Autodesk Inventor part; units mm, degrees
(part 3 of 5)
  line L98 (0, 22) -> (0, -22) construction
  circle A131 centre (-90.3659, 45.1111) radius 1.6
  circle A132 centre (-45.1111, 90.3659) radius 1.6
  circle A133 centre (90.3659, -45.1111) radius 1.6
  circle A134 centre (45.1111, -90.3659) radius 1.6
  circle A135 centre (90.3659, 45.1111) radius 1.6
  circle A136 centre (45.1111, 90.3659) radius 1.6
  line L99 (41.3657, 27.2236) -> (27.2236, 41.3657) construction
  line L100 (34.2947, 34.2947) -> (55.1543, 55.1543) construction
  line L101 (46.669, 63.6396) -> (63.6396, 46.669) construction
  line L102 (0, 0) -> (0, -61.2072) construction
  circle A137 centre (0, -54) radius 1.6
  arc A138 (3.4868, -52.0398) -> (-3.4868, -52.0398) centre (0, -54) ccw
  line L103 (-0.6161, -51.9466) -> (-14.5119, -56.4463) construction
  line L104 (-5.1776, -53.4237) -> (-14.5119, -56.4463) construction
  line L105 (14.5119, -56.4463) -> (0.6161, -51.9466) construction
  line L106 (5.1776, -53.4237) -> (14.5119, -56.4463) construction
  arc A139 (0, -58) -> (3.8733, -53.0013) centre (0, -54) ccw construction
  arc A140 (-3.8733, -53.0013) -> (0, -58) centre (0, -54) ccw construction
  arc A141 (-5.1776, -53.4237) -> (-3.4868, -52.0398) centre (-6.1018, -50.5696) ccw
  arc A142 (3.4868, -52.0398) -> (5.1776, -53.4237) centre (6.1018, -50.5696) ccw
  line L107 (5.1776, -53.4237) -> (3.794, -57.2809)
  line L108 (3.794, -57.2809) -> (-2.6441, -58)
  line L109 (-2.6441, -58) -> (-5.1776, -53.4237)
  dimension "d114" = 3.2
  dimension "d117" = 64
  dimension "d118" = 3.2
  dimension "d119" = 54
  dimension "d120" = 8
  dimension "d121" = 3
  constraints: 20 end point, 15 centre point, 14 point on circle, 7 symmetric about line, 6 point on line, 4 midpoint, 4 tangent, 2 coincident, 2 collinear, 2 vertical, 1 equal radius, 1 horizontal, 7 other
  measures "d114" diameter of A129
  measures "d117" distance of A135.centre A136.centre
  measures "d118" diameter of A137
  measures "d119" distance of A137.centre point (0, 0)
  measures "d120" diameter of A138
  measures "d121" radius of A141
extrude "Выдавливание9" cut sketch "Эскиз6" against normal blind 10 contours A129 | A130 | A131 | A132 | A133 | A134 | A135 | A136 | A137
extrude "Выдавливание10" add sketch "Эскиз6" against normal blind 2 contours A142 L107 L108 L109 A141 A138
sketch "Эскиз7" plane through (0, 2, 0) normal (0, 1, 0) x (1, 0, 0)
  line L0 (-25, -33.1335) -> (25, -33.1335) construction
  line L1 (25, -33.1335) -> (25, -43.1335) construction
  line L2 (25, -43.1335) -> (-25, -43.1335) construction
  line L3 (-25, -43.1335) -> (-25, -33.1335) construction
  line L4 (0, 0) -> (0, -69.4501) construction
  circle A0 centre (21.9203, -43.1335) radius 1.6 construction
  circle A1 centre (-21.9203, -43.1335) radius 1.6 construction
  dimension "d124" = 50
  dimension "d125" = 10
  constraints: 10 end point, 2 parallel, 1 horizontal, 1 perpendicular, 1 point on line, 1 vertical, 1 other
  measures "d124" distance of L1.end L2.end
  measures "d125" distance of L0.end L1.end
sketch "Эскиз8" plane through (0, 0, 0) normal (0, -1, 0) x (1, 0, 0)
  circle A0 centre (0, 54) radius 1.6 construction
  line L0 (14.5119, 56.4463) -> (5.1776, 53.4237) construction
  arc A1 (15.1585, 56.5907) -> (14.5119, 56.4463) centre (15.6055, 53.069) ccw construction
  line L1 (20.596, 57.2809) -> (15.1585, 56.5907) construction
  line L2 (20.596, 57.2809) -> (26.2105, 51.6664) construction
  line L3 (26.2105, 51.6664) -> (21.6698, 47.1257) construction
  arc A2 (21.6698, 47.1257) -> (17.9282, 43.384) centre (21.9203, 43.1335) ccw construction
  line L4 (17.9282, 43.384) -> (1.4142, 26.8701) construction
  arc A3 (-1.4142, 26.8701) -> (1.4142, 26.8701) centre (0, 28.2843) ccw construction
  line L5 (-1.4142, 26.8701) -> (-17.9282, 43.384) construction
  arc A4 (-17.9282, 43.384) -> (-21.6698, 47.1257) centre (-21.9203, 43.1335) ccw construction
  line L6 (-21.6698, 47.1257) -> (-26.2105, 51.6664) construction
  line L7 (-26.2105, 51.6664) -> (-20.596, 57.2809) construction
  line L8 (-15.1585, 56.5907) -> (-20.596, 57.2809) construction
  arc A5 (-14.5119, 56.4463) -> (-15.1585, 56.5907) centre (-15.6055, 53.069) ccw construction
  line L9 (-5.1776, 53.4237) -> (-14.5119, 56.4463) construction
  arc A6 (-3.4868, 52.0398) -> (-5.1776, 53.4237) centre (-6.1018, 50.5696) ccw construction
  arc A7 (-3.4868, 52.0398) -> (3.4868, 52.0398) centre (0, 54) ccw construction
  arc A8 (5.1776, 53.4237) -> (3.4868, 52.0398) centre (6.1018, 50.5696) ccw construction
  circle A9 centre (45.1111, 90.3659) radius 1.6 construction
  circle A10 centre (-45.1111, -90.3659) radius 1.6 construction
  circle A11 centre (-90.3659, -45.1111) radius 1.6 construction
  circle A12 centre (90.3659, 45.1111) radius 1.6 construction
  circle A13 centre (-45.1111, 90.3659) radius 1.6 construction
  circle A14 centre (45.1111, -90.3659) radius 1.6 construction
  circle A15 centre (-90.3659, 45.1111) radius 1.6 construction
  circle A16 centre (90.3659, -45.1111) radius 1.6 construction
  circle A17 centre (101, 0) radius 1.6 construction
  circle A18 centre (-101, 0) radius 1.6 construction
  arc A19 (-93.0503, 48.6481) -> (-93.0503, -48.6481) centre (0, 0) ccw construction
  arc A20 (-93.0503, -48.6481) -> (-88.2704, -49.3795) centre (-90.3917, -47.2582) ccw construction
  line L10 (-85.2064, -46.3155) -> (-88.2704, -49.3795) construction
  arc A21 (-73.8927, -46.3155) -> (-85.2064, -46.3155) centre (-79.5495, -51.9723) ccw construction
  line L11 (-46.3155, -73.8927) -> (-73.8927, -46.3155) construction
  arc A22 (-46.3155, -85.2064) -> (-46.3155, -73.8927) centre (-51.9723, -79.5495) ccw construction
  line L12 (-49.3795, -88.2704) -> (-46.3155, -85.2064) construction
  arc A23 (-49.3795, -88.2704) -> (-48.6481, -93.0503) centre (-47.2582, -90.3917) ccw construction
  arc A24 (-48.6481, -93.0503) -> (-11.8382, -104.3305) centre (0, 0) ccw construction
  arc A25 (-11.8382, -104.3305) -> (-8.5, -101.3496) centre (-11.5, -101.3496) ccw construction
  line L13 (-8.5, -101.3496) -> (-8.5, -90.5) construction
  arc A26 (-7, -89) -> (-8.5, -90.5) centre (-7, -90.5) ccw construction
  line L14 (-7, -89) -> (7, -89) construction
  arc A27 (8.5, -90.5) -> (7, -89) centre (7, -90.5) ccw construction
  line L15 (8.5, -90.5) -> (8.5, -101.3496) construction
  arc A28 (8.5, -101.3496) -> (11.8382, -104.3305) centre (11.5, -101.3496) ccw construction
  arc A29 (11.8382, -104.3305) -> (48.6481, -93.0503) centre (0, 0) ccw construction
  arc A30 (48.6481, -93.0503) -> (49.3795, -88.2704) centre (47.2582, -90.3917) ccw construction
  line L16 (46.3155, -85.2064) -> (49.3795, -88.2704) construction
  arc A31 (46.3155, -73.8927) -> (46.3155, -85.2064) centre (51.9723, -79.5495) ccw construction
  line L17 (73.8927, -46.3155) -> (46.3155, -73.8927) construction
  arc A32 (85.2064, -46.3155) -> (73.8927, -46.3155) centre (79.5495, -51.9723) ccw construction
  line L18 (88.2704, -49.3795) -> (85.2064, -46.3155) construction
  arc A33 (88.2704, -49.3795) -> (93.0503, -48.6481) centre (90.3917, -47.2582) ccw construction
  arc A34 (93.0503, -48.6481) -> (93.0503, 48.6481) centre (0, 0) ccw construction
  arc A35 (93.0503, 48.6481) -> (88.2704, 49.3795) centre (90.3917, 47.2582) ccw construction
  line L19 (85.2064, 46.3155) -> (88.2704, 49.3795) construction
  arc A36 (73.8927, 46.3155) -> (85.2064, 46.3155) centre (79.5495, 51.9723) ccw construction
  line L20 (46.3155, 73.8927) -> (73.8927, 46.3155) construction
  arc A37 (46.3155, 85.2064) -> (46.3155, 73.8927) centre (51.9723, 79.5495) ccw construction
  line L21 (49.3795, 88.2704) -> (46.3155, 85.2064) construction
  arc A38 (49.3795, 88.2704) -> (48.6481, 93.0503) centre (47.2582, 90.3917) ccw construction
  arc A39 (48.6481, 93.0503) -> (45.42, 94.668) centre (0, 0) ccw construction
  arc A40 (45.42, 94.668) -> (43.0355, 94.1655) centre (44.5548, 92.8648) ccw construction
  line L22 (18.3802, 65.3664) -> (43.0355, 94.1655) construction
  arc A41 (17.477, 64.7643) -> (18.3802, 65.3664) centre (16.8609, 66.6671) ccw construction
  line L23 (0.6161, 59.3045) -> (17.477, 64.7643) construction
  arc A42 (-0.6161, 59.3045) -> (0.6161, 59.3045) centre (0, 61.2072) ccw construction
  line L24 (-17.477, 64.7643) -> (-0.6161, 59.3045) construction
  arc A43 (-18.3802, 65.3664) -> (-17.477, 64.7643) centre (-16.8609, 66.6671) ccw construction
  line L25 (-43.0355, 94.1655) -> (-18.3802, 65.3664) construction
  arc A44 (-43.0355, 94.1655) -> (-45.42, 94.668) centre (-44.5548, 92.8648) ccw construction
  arc A45 (-45.42, 94.668) -> (-48.6481, 93.0503) centre (0, 0) ccw construction
  arc A46 (-48.6481, 93.0503) -> (-49.3795, 88.2704) centre (-47.2582, 90.3917) ccw construction
  line L26 (-46.3155, 85.2064) -> (-49.3795, 88.2704) construction
  arc A47 (-46.3155, 73.8927) -> (-46.3155, 85.2064) centre (-51.9723, 79.5495) ccw construction
  line L27 (-73.8927, 46.3155) -> (-46.3155, 73.8927) construction
  arc A48 (-85.2064, 46.3155) -> (-73.8927, 46.3155) centre (-79.5495, 51.9723) ccw construction
  line L28 (-88.2704, 49.3795) -> (-85.2064, 46.3155) construction
  arc A49 (-88.2704, 49.3795) -> (-93.0503, 48.6481) centre (-90.3917, 47.2582) ccw construction
  arc A50 (90.4395, -37.7453) -> (97.9653, -2.6059) centre (0, 0) ccw construction
  arc A51 (87.1795, -38.3892) -> (90.4395, -37.7453) centre (88.5938, -36.975) ccw construction
  line L29 (83.085, -34.2947) -> (87.1795, -38.3892) construction
  arc A52 (83.085, -34.2947) -> (76.014, -34.2947) centre (79.5495, -37.8302) ccw construction
  line L30 (67.8823, -42.4264) -> (76.014, -34.2947) construction
  line L31 (67.8823, -42.4264) -> (47.1257, -21.6698) construction
  arc A53 (47.1257, -21.6698) -> (43.384, -17.9282) centre (43.1335, -21.9203) ccw construction
  line L32 (43.384, -17.9282) -> (26.8701, -1.4142) construction
  arc A54 (26.8701, 1.4142) -> (26.8701, -1.4142) centre (28.2843, 0) ccw construction
  line L33 (26.8701, 1.4142) -> (43.384, 17.9282) construction
  arc A55 (43.384, 17.9282) -> (47.1257, 21.6698) centre (43.1335, 21.9203) ccw construction
  line L34 (47.1257, 21.6698) -> (67.8823, 42.4264) construction
  line L35 (76.014, 34.2947) -> (67.8823, 42.4264) construction
  arc A56 (76.014, 34.2947) -> (83.085, 34.2947) centre (79.5495, 37.8302) ccw construction
  line L36 (87.1795, 38.3892) -> (83.085, 34.2947) construction
  arc A57 (90.4395, 37.7453) -> (87.1795, 38.3892) centre (88.5938, 36.975) ccw construction
  arc A58 (97.9653, 2.6059) -> (90.4395, 37.7453) centre (0, 0) ccw construction
  arc A59 (97.9653, 2.6059) -> (97.9653, -2.6059) centre (101, 0) ccw construction
  line L37 (29.746, 55.2019) -> (24.3148, 60.6331) construction
  line L38 (24.842, 61.8893) -> (24.3148, 60.6331) construction
  arc A60 (25.4187, 62.8242) -> (24.842, 61.8893) centre (28.1154, 60.5155) ccw construction
  line L39 (34.1909, 73.0707) -> (25.4187, 62.8242) construction
  arc A61 (37.1244, 73.1843) -> (34.1909, 73.0707) centre (35.7102, 71.7701) ccw construction
  line L40 (42.4264, 67.8823) -> (37.1244, 73.1843) construction
  line L41 (42.4264, 67.8823) -> (29.746, 55.2019) construction
  arc A62 (14.5, -93.3742) -> (18.0526, -96.3229) centre (17.5, -93.3742) ccw construction
  line L42 (14.5, -93.3742) -> (14.5, -87) construction
  arc A63 (14.5, -87) -> (11.5, -84) centre (11.5, -87) ccw construction
  line L43 (11.5, -84) -> (-11.5, -84) construction
  arc A64 (-11.5, -84) -> (-14.5, -87) centre (-11.5, -87) ccw construction
  line L44 (-14.5, -87) -> (-14.5, -93.3742) construction
  arc A65 (-18.0526, -96.3229) -> (-14.5, -93.3742) centre (-17.5, -93.3742) ccw construction
  arc A66 (-37.7453, -90.4395) -> (-18.0526, -96.3229) centre (0, 0) ccw construction
  arc A67 (-38.3892, -87.1795) -> (-37.7453, -90.4395) centre (-36.975, -88.5938) ccw construction
  line L45 (-34.2947, -83.085) -> (-38.3892, -87.1795) construction
  arc A68 (-34.2947, -83.085) -> (-34.2947, -76.014) centre (-37.8302, -79.5495) ccw construction
  line L46 (-42.4264, -67.8823) -> (-34.2947, -76.014) construction
  line L47 (-42.4264, -67.8823) -> (-21.6698, -47.1257) construction
  arc A69 (-21.6698, -47.1257) -> (-17.9282, -43.384) centre (-21.9203, -43.1335) ccw construction
  line L48 (-17.9282, -43.384) -> (-1.4142, -26.8701) construction
  arc A70 (1.4142, -26.8701) -> (-1.4142, -26.8701) centre (0, -28.2843) ccw construction
  line L49 (1.4142, -26.8701) -> (17.9282, -43.384) construction
  arc A71 (17.9282, -43.384) -> (21.6698, -47.1257) centre (21.9203, -43.1335) ccw construction
  line L50 (21.6698, -47.1257) -> (42.4264, -67.8823) construction
  line L51 (34.2947, -76.014) -> (42.4264, -67.8823) construction
  arc A72 (34.2947, -76.014) -> (34.2947, -83.085) centre (37.8302, -79.5495) ccw construction
  line L52 (38.3892, -87.1795) -> (34.2947, -83.085) construction
  arc A73 (37.7453, -90.4395) -> (38.3892, -87.1795) centre (36.975, -88.5938) ccw construction
  arc A74 (18.0526, -96.3229) -> (37.7453, -90.4395) centre (0, 0) ccw construction
  line L53 (63.6396, 46.669) -> (46.669, 63.6396) construction
  line L54 (63.6396, 46.669) -> (44.1942, 27.2236) construction
  arc A75 (41.3657, 27.2236) -> (44.1942, 27.2236) centre (42.78, 28.6378) ccw construction
  line L55 (41.3657, 27.2236) -> (27.2236, 41.3657) construction
  arc A76 (27.2236, 44.1942) -> (27.2236, 41.3657) centre (28.6378, 42.78) ccw construction
  line L56 (27.2236, 44.1942) -> (46.669, 63.6396) construction
  line L57 (46.669, -63.6396) -> (63.6396, -46.669) construction
  line L58 (46.669, -63.6396) -> (27.2236, -44.1942) construction
  arc A77 (27.2236, -41.3657) -> (27.2236, -44.1942) centre (28.6378, -42.78) ccw construction
  line L59 (27.2236, -41.3657) -> (41.3657, -27.2236) construction
  arc A78 (44.1942, -27.2236) -> (41.3657, -27.2236) centre (42.78, -28.6378) ccw construction
  line L60 (44.1942, -27.2236) -> (63.6396, -46.669) construction
  line L61 (-63.6396, -46.669) -> (-46.669, -63.6396) construction
  line L62 (-63.6396, -46.669) -> (-44.1942, -27.2236) construction
  arc A79 (-41.3657, -27.2236) -> (-44.1942, -27.2236) centre (-42.78, -28.6378) ccw construction
  line L63 (-41.3657, -27.2236) -> (-27.2236, -41.3657) construction
  arc A80 (-27.2236, -44.1942) -> (-27.2236, -41.3657) centre (-28.6378, -42.78) ccw construction
  line L64 (-27.2236, -44.1942) -> (-46.669, -63.6396) construction
  line L65 (-46.669, 63.6396) -> (-63.6396, 46.669) construction
  line L66 (-46.669, 63.6396) -> (-27.2236, 44.1942) construction
  arc A81 (-27.2236, 41.3657) -> (-27.2236, 44.1942) centre (-28.6378, 42.78) ccw construction
  line L67 (-27.2236, 41.3657) -> (-41.3657, 27.2236) construction
  arc A82 (-44.1942, 27.2236) -> (-41.3657, 27.2236) centre (-42.78, 28.6378) ccw construction
  line L68 (-44.1942, 27.2236) -> (-63.6396, 46.669) construction
  arc A83 (7.7166, 24.6871) -> (8.4003, 21.4111) centre (9.1308, 23.2729) ccw construction
  line L69 (7.7166, 24.6871) -> (20.8597, 37.8302) construction
  arc A84 (23.6881, 37.8302) -> (20.8597, 37.8302) centre (22.2739, 36.416) ccw construction
  line L70 (23.6881, 37.8302) -> (37.8302, 23.6881) construction
  arc A85 (37.8302, 20.8597) -> (37.8302, 23.6881) centre (36.416, 22.2739) ccw construction
  line L71 (37.8302, 20.8597) -> (24.6871, 7.7166) construction
  arc A86 (21.4111, 8.4003) -> (24.6871, 7.7166) centre (23.2729, 9.1308) ccw construction
  arc A87 (21.4111, 8.4003) -> (8.4003, 21.4111) centre (0, 0) ccw construction
  circle A88 centre (-21.9203, -43.1335) radius 1.6 construction
  arc A89 (-21.4111, -8.4003) -> (-24.6871, -7.7166) centre (-23.2729, -9.1308) ccw construction
  arc A90 (-21.4111, -8.4003) -> (-8.4003, -21.4111) centre (0, 0) ccw construction
  arc A91 (-7.7166, -24.6871) -> (-8.4003, -21.4111) centre (-9.1308, -23.2729) ccw construction
  line L72 (-7.7166, -24.6871) -> (-20.8597, -37.8302) construction
  arc A92 (-23.6881, -37.8302) -> (-20.8597, -37.8302) centre (-22.2739, -36.416) ccw construction
  line L73 (-23.6881, -37.8302) -> (-37.8302, -23.6881) construction
  arc A93 (-37.8302, -20.8597) -> (-37.8302, -23.6881) centre (-36.416, -22.2739) ccw construction
  line L74 (-37.8302, -20.8597) -> (-24.6871, -7.7166) construction
  line L75 (24.6871, -7.7166) -> (37.8302, -20.8597) construction
  arc A94 (37.8302, -23.6881) -> (37.8302, -20.8597) centre (36.416, -22.2739) ccw construction
  line L76 (37.8302, -23.6881) -> (23.6881, -37.8302) construction
  arc A95 (20.8597, -37.8302) -> (23.6881, -37.8302) centre (22.2739, -36.416) ccw construction
  line L77 (20.8597, -37.8302) -> (7.7166, -24.6871) construction
  arc A96 (8.4003, -21.4111) -> (7.7166, -24.6871) centre (9.1308, -23.2729) ccw construction
  arc A97 (8.4003, -21.4111) -> (21.4111, -8.4003) centre (0, 0) ccw construction
  arc A98 (24.6871, -7.7166) -> (21.4111, -8.4003) centre (23.2729, -9.1308) ccw construction
  circle A99 centre (21.9203, 43.1335) radius 1.6 construction
  line L78 (-37.8302, 23.6881) -> (-23.6881, 37.8302) construction
  arc A100 (-20.8597, 37.8302) -> (-23.6881, 37.8302) centre (-22.2739, 36.416) ccw construction
  line L79 (-20.8597, 37.8302) -> (-7.7166, 24.6871) construction
  arc A101 (-8.4003, 21.4111) -> (-7.7166, 24.6871) centre (-9.1308, 23.2729) ccw construction
  arc A102 (-8.4003, 21.4111) -> (-21.4111, 8.4003) centre (0, 0) ccw construction
  arc A103 (-24.6871, 7.7166) -> (-21.4111, 8.4003) centre (-23.2729, 9.1308) ccw construction
  line L80 (-24.6871, 7.7166) -> (-37.8302, 20.8597) construction
  arc A104 (-37.8302, 23.6881) -> (-37.8302, 20.8597) centre (-36.416, 22.2739) ccw construction
  circle A105 centre (-43.1335, 21.9203) radius 1.6 construction
  circle A106 centre (43.1335, -21.9203) radius 1.6 construction
  circle A107 centre (21.9203, -43.1335) radius 1.6 construction
  circle A108 centre (-21.9203, 43.1335) radius 1.6 construction
  circle A109 centre (-43.1335, -21.9203) radius 1.6 construction
  circle A110 centre (0, 0) radius 18 construction
  circle A111 centre (43.1335, 21.9203) radius 1.6 construction
  circle A112 centre (0, -22) radius 1.6 construction
  circle A113 centre (-22, 0) radius 1.6 construction
  circle A114 centre (0, 22) radius 1.6 construction
  circle A115 centre (22, 0) radius 1.6 construction
  circle A116 centre (-37.8302, -79.5495) radius 1.6 construction
  circle A117 centre (-79.5495, -37.8302) radius 1.6 construction
  circle A118 centre (-79.5495, 37.8302) radius 1.6 construction
  circle A119 centre (79.5495, 37.8302) radius 1.6 construction
  circle A120 centre (37.8302, -79.5495) radius 1.6 construction
  circle A121 centre (79.5495, -37.8302) radius 1.6 construction
  circle A122 centre (-20.5578, 60.8546) radius 1.55 construction
  circle A123 centre (20.5578, 60.8546) radius 1.55 construction
  circle A124 centre (37.8302, 79.5495) radius 1.6 construction
  circle A125 centre (-37.8302, 79.5495) radius 1.6 construction
  line L81 (-24.3148, 60.6331) -> (-29.746, 55.2019) construction
  line L82 (-29.746, 55.2019) -> (-42.4264, 67.8823) construction
  line L83 (-37.1244, 73.1843) -> (-42.4264, 67.8823) construction
  arc A126 (-34.1909, 73.0707) -> (-37.1244, 73.1843) centre (-35.7102, 71.7701) ccw construction
  line L84 (-25.4187, 62.8242) -> (-34.1909, 73.0707) construction
  arc A127 (-24.842, 61.8893) -> (-25.4187, 62.8242) centre (-28.1154, 60.5155) ccw construction
  line L85 (-24.3148, 60.6331) -> (-24.842, 61.8893) construction
  arc A128 (-90.4395, 37.7453) -> (-97.9653, 2.6059) centre (0, 0) ccw construction
  arc A129 (-87.1795, 38.3892) -> (-90.4395, 37.7453) centre (-88.5938, 36.975) ccw construction
  line L86 (-83.085, 34.2947) -> (-87.1795, 38.3892) construction
  arc A130 (-83.085, 34.2947) -> (-76.014, 34.2947) centre (-79.5495, 37.8302) ccw construction
  line L87 (-67.8823, 42.4264) -> (-76.014, 34.2947) construction
  line L88 (-67.8823, 42.4264) -> (-47.1257, 21.6698) construction
  arc A131 (-47.1257, 21.6698) -> (-43.384, 17.9282) centre (-43.1335, 21.9203) ccw construction
  line L89 (-43.384, 17.9282) -> (-26.8701, 1.4142) construction
  arc A132 (-26.8701, -1.4142) -> (-26.8701, 1.4142) centre (-28.2843, 0) ccw construction
  line L90 (-26.8701, -1.4142) -> (-43.384, -17.9282) construction
  arc A133 (-43.384, -17.9282) -> (-47.1257, -21.6698) centre (-43.1335, -21.9203) ccw construction
  line L91 (-47.1257, -21.6698) -> (-67.8823, -42.4264) construction
  line L92 (-76.014, -34.2947) -> (-67.8823, -42.4264) construction
  arc A134 (-76.014, -34.2947) -> (-83.085, -34.2947) centre (-79.5495, -37.8302) ccw construction
  line L93 (-87.1795, -38.3892) -> (-83.085, -34.2947) construction
  arc A135 (-90.4395, -37.7453) -> (-87.1795, -38.3892) centre (-88.5938, -36.975) ccw construction
  arc A136 (-97.9653, -2.6059) -> (-90.4395, -37.7453) centre (0, 0) ccw construction
  arc A137 (-97.9653, -2.6059) -> (-97.9653, 2.6059) centre (-101, 0) ccw construction
  line L94 (19.5177, 122.3748) -> (96.2153, 45.6773) construction
  arc A138 (93.0503, 48.6481) -> (88.2704, 49.3795) centre (90.3917, 47.2582) ccw construction
  line L95 (-105.344, -36.5485) -> (-36.5776, -105.315) construction
  arc A139 (-49.3795, -88.2704) -> (-48.6481, -93.0503) centre (-47.2582, -90.3917) ccw construction
  arc A140 (-93.0503, -48.6481) -> (-88.2704, -49.3795) centre (-90.3917, -47.2582) ccw construction
  circle A141 centre (0, 54) radius 1.6 construction
  arc A142 (-93.0503, 48.6481) -> (-93.0503, -48.6481) centre (0, 0) ccw construction
  arc A143 (-88.2704, 49.3795) -> (-93.0503, 48.6481) centre (-90.3917, 47.2582) ccw construction
  line L96 (-88.2704, 49.3795) -> (-85.2064, 46.3155) construction
  arc A144 (-85.2064, 46.3155) -> (-73.8927, 46.3155) centre (-79.5495, 51.9723) ccw construction
  line L97 (-73.8927, 46.3155) -> (-46.3155, 73.8927) construction
  arc A145 (-46.3155, 73.8927) -> (-46.3155, 85.2064) centre (-51.9723, 79.5495) ccw construction
  line L98 (-46.3155, 85.2064) -> (-49.3795, 88.2704) construction
  arc A146 (-48.6481, 93.0503) -> (-49.3795, 88.2704) centre (-47.2582, 90.3917) ccw construction
  arc A147 (-45.42, 94.668) -> (-48.6481, 93.0503) centre (0, 0) ccw construction
  arc A148 (-43.0355, 94.1655) -> (-45.42, 94.668) centre (-44.5548, 92.8648) ccw construction
  line L99 (-43.0355, 94.1655) -> (-18.3802, 65.3664) construction
  arc A149 (-18.3802, 65.3664) -> (-17.477, 64.7643) centre (-16.8609, 66.6671) ccw construction
  line L100 (-17.477, 64.7643) -> (-0.6161, 59.3045) construction
  arc A150 (-0.6161, 59.3045) -> (0.6161, 59.3045) centre (0, 61.2072) ccw construction
  line L101 (0.6161, 59.3045) -> (17.477, 64.7643) construction
  arc A151 (17.477, 64.7643) -> (18.3802, 65.3664) centre (16.8609, 66.6671) ccw construction
  line L102 (18.3802, 65.3664) -> (43.0355, 94.1655) construction
  arc A152 (45.42, 94.668) -> (43.0355, 94.1655) centre (44.5548, 92.8648) ccw construction
  arc A153 (48.6481, 93.0503) -> (45.42, 94.668) centre (0, 0) ccw construction
  arc A154 (49.3795, 88.2704) -> (48.6481, 93.0503) centre (47.2582, 90.3917) ccw construction
  line L103 (49.3795, 88.2704) -> (46.3155, 85.2064) construction
  arc A155 (46.3155, 85.2064) -> (46.3155, 73.8927) centre (51.9723, 79.5495) ccw construction
  line L104 (46.3155, 73.8927) -> (73.8927, 46.3155) construction
  arc A156 (73.8927, 46.3155) -> (85.2064, 46.3155) centre (79.5495, 51.9723) ccw construction
  line L105 (85.2064, 46.3155) -> (88.2704, 49.3795) construction
  arc A157 (93.0503, 48.6481) -> (88.2704, 49.3795) centre (90.3917, 47.2582) ccw construction
  arc A158 (93.0503, -48.6481) -> (93.0503, 48.6481) centre (0, 0) ccw construction
  arc A159 (88.2704, -49.3795) -> (93.0503, -48.6481) centre (90.3917, -47.2582) ccw construction
  line L106 (88.2704, -49.3795) -> (85.2064, -46.3155) construction
  arc A160 (85.2064, -46.3155) -> (73.8927, -46.3155) centre (79.5495, -51.9723) ccw construction
  line L107 (73.8927, -46.3155) -> (46.3155, -73.8927) construction
  arc A161 (46.3155, -73.8927) -> (46.3155, -85.2064) centre (51.9723, -79.5495) ccw construction
  line L108 (46.3155, -85.2064) -> (49.3795, -88.2704) construction
  arc A162 (48.6481, -93.0503) -> (49.3795, -88.2704) centre (47.2582, -90.3917) ccw construction
  arc A163 (11.8382, -104.3305) -> (48.6481, -93.0503) centre (0, 0) ccw construction
  arc A164 (8.5, -101.3496) -> (11.8382, -104.3305) centre (11.5, -101.3496) ccw construction
  line L109 (8.5, -101.3496) -> (8.5, -90.5) construction
  arc A165 (8.5, -90.5) -> (7, -89) centre (7, -90.5) ccw construction
  line L110 (7, -89) -> (-7, -89) construction
  arc A166 (-7, -89) -> (-8.5, -90.5) centre (-7, -90.5) ccw construction
  line L111 (-8.5, -90.5) -> (-8.5, -101.3496) construction
  arc A167 (-11.8382, -104.3305) -> (-8.5, -101.3496) centre (-11.5, -101.3496) ccw construction
  arc A168 (-48.6481, -93.0503) -> (-11.8382, -104.3305) centre (0, 0) ccw construction
  arc A169 (-49.3795, -88.2704) -> (-48.6481, -93.0503) centre (-47.2582, -90.3917) ccw construction
  line L112 (-49.3795, -88.2704) -> (-46.3155, -85.2064) construction
  arc A170 (-46.3155, -85.2064) -> (-46.3155, -73.8927) centre (-51.9723, -79.5495) ccw construction
  line L113 (-46.3155, -73.8927) -> (-73.8927, -46.3155) construction
  arc A171 (-73.8927, -46.3155) -> (-85.2064, -46.3155) centre (-79.5495, -51.9723) ccw construction
  line L114 (-85.2064, -46.3155) -> (-88.2704, -49.3795) construction
  arc A172 (-93.0503, -48.6481) -> (-88.2704, -49.3795) centre (-90.3917, -47.2582) ccw construction
  arc A173 (-97.9653, -2.6059) -> (-90.4395, -37.7453) centre (0, 0) ccw construction
  arc A174 (-90.4395, -37.7453) -> (-87.1795, -38.3892) centre (-88.5938, -36.975) ccw construction
  line L115 (-87.1795, -38.3892) -> (-83.085, -34.2947) construction
  arc A175 (-76.014, -34.2947) -> (-83.085, -34.2947) centre (-79.5495, -37.8302) ccw construction
  line L116 (-76.014, -34.2947) -> (-67.8823, -42.4264) construction
  line L117 (-67.8823, -42.4264) -> (-47.1257, -21.6698) construction
  arc A176 (-43.384, -17.9282) -> (-47.1257, -21.6698) centre (-43.1335, -21.9203) ccw construction
  line L118 (-43.384, -17.9282) -> (-26.8701, -1.4142) construction
  arc A177 (-26.8701, -1.4142) -> (-26.8701, 1.4142) centre (-28.2843, 0) ccw construction
  line L119 (-26.8701, 1.4142) -> (-43.384, 17.9282) construction
  arc A178 (-47.1257, 21.6698) -> (-43.384, 17.9282) centre (-43.1335, 21.9203) ccw construction
  line L120 (-47.1257, 21.6698) -> (-67.8823, 42.4264) construction
  line L121 (-67.8823, 42.4264) -> (-76.014, 34.2947) construction
  arc A179 (-83.085, 34.2947) -> (-76.014, 34.2947) centre (-79.5495, 37.8302) ccw construction
  line L122 (-83.085, 34.2947) -> (-87.1795, 38.3892) construction
  arc A180 (-87.1795, 38.3892) -> (-90.4395, 37.7453) centre (-88.5938, 36.975) ccw construction
  arc A181 (-90.4395, 37.7453) -> (-97.9653, 2.6059) centre (0, 0) ccw construction
  arc A182 (-97.9653, -2.6059) -> (-97.9653, 2.6059) centre (-101, 0) ccw construction
  line L123 (29.746, 55.2019) -> (42.4264, 67.8823) construction
  line L124 (42.4264, 67.8823) -> (37.1244, 73.1843) construction
  arc A183 (37.1244, 73.1843) -> (34.1909, 73.0707) centre (35.7102, 71.7701) ccw construction
  line L125 (34.1909, 73.0707) -> (25.4187, 62.8242) construction
  arc A184 (25.4187, 62.8242) -> (24.842, 61.8893) centre (28.1154, 60.5155) ccw construction
  line L126 (24.842, 61.8893) -> (24.3148, 60.6331) construction
  line L127 (24.3148, 60.6331) -> (29.746, 55.2019) construction
  arc A185 (5.1776, 53.4237) -> (3.4868, 52.0398) centre (6.1018, 50.5696) ccw construction
  arc A186 (-3.4868, 52.0398) -> (3.4868, 52.0398) centre (0, 54) ccw construction
  arc A187 (-3.4868, 52.0398) -> (-5.1776, 53.4237) centre (-6.1018, 50.5696) ccw construction
  line L128 (-5.1776, 53.4237) -> (-14.5119, 56.4463) construction
  arc A188 (-14.5119, 56.4463) -> (-15.1585, 56.5907) centre (-15.6055, 53.069) ccw construction
  line L129 (-15.1585, 56.5907) -> (-20.596, 57.2809) construction
  line L130 (-20.596, 57.2809) -> (-26.2105, 51.6664) construction
  line L131 (-26.2105, 51.6664) -> (-21.6698, 47.1257) construction
  arc A189 (-17.9282, 43.384) -> (-21.6698, 47.1257) centre (-21.9203, 43.1335) ccw construction
  line L132 (-17.9282, 43.384) -> (-1.4142, 26.8701) construction
  arc A190 (-1.4142, 26.8701) -> (1.4142, 26.8701) centre (0, 28.2843) ccw construction
  line L133 (1.4142, 26.8701) -> (17.9282, 43.384) construction
  arc A191 (21.6698, 47.1257) -> (17.9282, 43.384) centre (21.9203, 43.1335) ccw construction
  line L134 (21.6698, 47.1257) -> (26.2105, 51.6664) construction
  line L135 (26.2105, 51.6664) -> (20.596, 57.2809) construction
  line L136 (20.596, 57.2809) -> (15.1585, 56.5907) construction
  arc A192 (15.1585, 56.5907) -> (14.5119, 56.4463) centre (15.6055, 53.069) ccw construction
  line L137 (14.5119, 56.4463) -> (5.1776, 53.4237) construction
  arc A193 (18.0526, -96.3229) -> (37.7453, -90.4395) centre (0, 0) ccw construction
  arc A194 (37.7453, -90.4395) -> (38.3892, -87.1795) centre (36.975, -88.5938) ccw construction
  line L138 (38.3892, -87.1795) -> (34.2947, -83.085) construction
  arc A195 (34.2947, -76.014) -> (34.2947, -83.085) centre (37.8302, -79.5495) ccw construction
  line L139 (34.2947, -76.014) -> (42.4264, -67.8823) construction
  line L140 (42.4264, -67.8823) -> (21.6698, -47.1257) construction
  arc A196 (17.9282, -43.384) -> (21.6698, -47.1257) centre (21.9203, -43.1335) ccw construction
  line L141 (17.9282, -43.384) -> (1.4142, -26.8701) construction
  arc A197 (1.4142, -26.8701) -> (-1.4142, -26.8701) centre (0, -28.2843) ccw construction
  line L142 (-1.4142, -26.8701) -> (-17.9282, -43.384) construction
  arc A198 (-21.6698, -47.1257) -> (-17.9282, -43.384) centre (-21.9203, -43.1335) ccw construction
  line L143 (-21.6698, -47.1257) -> (-42.4264, -67.8823) construction
  line L144 (-42.4264, -67.8823) -> (-34.2947, -76.014) construction
  arc A199 (-34.2947, -83.085) -> (-34.2947, -76.014) centre (-37.8302, -79.5495) ccw construction
  line L145 (-34.2947, -83.085) -> (-38.3892, -87.1795) construction
  arc A200 (-38.3892, -87.1795) -> (-37.7453, -90.4395) centre (-36.975, -88.5938) ccw construction
  arc A201 (-37.7453, -90.4395) -> (-18.0526, -96.3229) centre (0, 0) ccw construction
  arc A202 (-18.0526, -96.3229) -> (-14.5, -93.3742) centre (-17.5, -93.3742) ccw construction
  line L146 (-14.5, -93.3742) -> (-14.5, -87) construction
  arc A203 (-11.5, -84) -> (-14.5, -87) centre (-11.5, -87) ccw construction
  line L147 (-11.5, -84) -> (11.5, -84) construction
  arc A204 (14.5, -87) -> (11.5, -84) centre (11.5, -87) ccw construction
  line L148 (14.5, -87) -> (14.5, -93.3742) construction
  arc A205 (14.5, -93.3742) -> (18.0526, -96.3229) centre (17.5, -93.3742) ccw construction
  line L149 (63.6396, -46.669) -> (44.1942, -27.2236) construction
  arc A206 (44.1942, -27.2236) -> (41.3657, -27.2236) centre (42.78, -28.6378) ccw construction
  line L150 (41.3657, -27.2236) -> (27.2236, -41.3657) construction
  arc A207 (27.2236, -41.3657) -> (27.2236, -44.1942) centre (28.6378, -42.78) ccw construction
  line L151 (27.2236, -44.1942) -> (46.669, -63.6396) construction
  line L152 (46.669, -63.6396) -> (63.6396, -46.669) construction
  circle A208 centre (-37.8302, 79.5495) radius 1.6 construction
  circle A209 centre (37.8302, 79.5495) radius 1.6 construction
  circle A210 centre (20.5578, 60.8546) radius 1.55 construction
  circle A211 centre (-20.5578, 60.8546) radius 1.55 construction
  circle A212 centre (79.5495, -37.8302) radius 1.6 construction
  circle A213 centre (37.8302, -79.5495) radius 1.6 construction
  circle A214 centre (79.5495, 37.8302) radius 1.6 construction
  circle A215 centre (-79.5495, 37.8302) radius 1.6 construction
  circle A216 centre (-79.5495, -37.8302) radius 1.6 construction
  circle A217 centre (-37.8302, -79.5495) radius 1.6 construction
  circle A218 centre (22, 0) radius 1.6 construction
  circle A219 centre (0, 22) radius 1.6 construction
  circle A220 centre (-22, 0) radius 1.6 construction
  circle A221 centre (0, -22) radius 1.6 construction
  circle A222 centre (43.1335, 21.9203) radius 1.6 construction
  circle A223 centre (0, 0) radius 18 construction
  circle A224 centre (-43.1335, -21.9203) radius 1.6 construction
  circle A225 centre (-21.9203, 43.1335) radius 1.6 construction
  circle A226 centre (21.9203, -43.1335) radius 1.6 construction
  circle A227 centre (43.1335, -21.9203) radius 1.6 construction
  circle A228 centre (-43.1335, 21.9203) radius 1.6 construction
  arc A229 (-37.8302, 23.6881) -> (-37.8302, 20.8597) centre (-36.416, 22.2739) ccw construction
  line L153 (-37.8302, 20.8597) -> (-24.6871, 7.7166) construction
  arc A230 (-24.6871, 7.7166) -> (-21.4111, 8.4003) centre (-23.2729, 9.1308) ccw construction
  arc A231 (-8.4003, 21.4111) -> (-21.4111, 8.4003) centre (0, 0) ccw construction
  arc A232 (-8.4003, 21.4111) -> (-7.7166, 24.6871) centre (-9.1308, 23.2729) ccw construction
  line L154 (-7.7166, 24.6871) -> (-20.8597, 37.8302) construction
  arc A233 (-20.8597, 37.8302) -> (-23.6881, 37.8302) centre (-22.2739, 36.416) ccw construction
  line L155 (-23.6881, 37.8302) -> (-37.8302, 23.6881) construction
  circle A234 centre (21.9203, 43.1335) radius 1.6 construction
  arc A235 (20.8597, -37.8302) -> (23.6881, -37.8302) centre (22.2739, -36.416) ccw construction
  line L156 (23.6881, -37.8302) -> (37.8302, -23.6881) construction
  arc A236 (37.8302, -23.6881) -> (37.8302, -20.8597) centre (36.416, -22.2739) ccw construction
  line L157 (37.8302, -20.8597) -> (24.6871, -7.7166) construction
  arc A237 (24.6871, -7.7166) -> (21.4111, -8.4003) centre (23.2729, -9.1308) ccw construction
  arc A238 (8.4003, -21.4111) -> (21.4111, -8.4003) centre (0, 0) ccw construction
  arc A239 (8.4003, -21.4111) -> (7.7166, -24.6871) centre (9.1308, -23.2729) ccw construction
  line L158 (7.7166, -24.6871) -> (20.8597, -37.8302) construction
  line L159 (-37.8302, -23.6881) -> (-23.6881, -37.8302) construction
  arc A240 (-23.6881, -37.8302) -> (-20.8597, -37.8302) centre (-22.2739, -36.416) ccw construction
  line L160 (-20.8597, -37.8302) -> (-7.7166, -24.6871) construction
  arc A241 (-7.7166, -24.6871) -> (-8.4003, -21.4111) centre (-9.1308, -23.2729) ccw construction
  arc A242 (-21.4111, -8.4003) -> (-8.4003, -21.4111) centre (0, 0) ccw construction
  arc A243 (-21.4111, -8.4003) -> (-24.6871, -7.7166) centre (-23.2729, -9.1308) ccw construction
  line L161 (-24.6871, -7.7166) -> (-37.8302, -20.8597) construction
  arc A244 (-37.8302, -20.8597) -> (-37.8302, -23.6881) centre (-36.416, -22.2739) ccw construction
  circle A245 centre (-21.9203, -43.1335) radius 1.6 construction
  line L162 (24.6871, 7.7166) -> (37.8302, 20.8597) construction
  arc A246 (37.8302, 20.8597) -> (37.8302, 23.6881) centre (36.416, 22.2739) ccw construction
  line L163 (37.8302, 23.6881) -> (23.6881, 37.8302) construction
  arc A247 (23.6881, 37.8302) -> (20.8597, 37.8302) centre (22.2739, 36.416) ccw construction
  line L164 (20.8597, 37.8302) -> (7.7166, 24.6871) construction
  arc A248 (7.7166, 24.6871) -> (8.4003, 21.4111) centre (9.1308, 23.2729) ccw construction
  arc A249 (21.4111, 8.4003) -> (8.4003, 21.4111) centre (0, 0) ccw construction
  arc A250 (21.4111, 8.4003) -> (24.6871, 7.7166) centre (23.2729, 9.1308) ccw construction
  line L165 (46.669, 63.6396) -> (27.2236, 44.1942) construction
  arc A251 (27.2236, 44.1942) -> (27.2236, 41.3657) centre (28.6378, 42.78) ccw construction
  line L166 (27.2236, 41.3657) -> (41.3657, 27.2236) construction
  arc A252 (41.3657, 27.2236) -> (44.1942, 27.2236) centre (42.78, 28.6378) ccw construction
  line L167 (44.1942, 27.2236) -> (63.6396, 46.669) construction
  line L168 (63.6396, 46.669) -> (46.669, 63.6396) construction
  line L169 (-29.746, 55.2019) -> (-24.3148, 60.6331) construction
  line L170 (-24.3148, 60.6331) -> (-24.842, 61.8893) construction
  arc A253 (-24.842, 61.8893) -> (-25.4187, 62.8242) centre (-28.1154, 60.5155) ccw construction
  line L171 (-25.4187, 62.8242) -> (-34.1909, 73.0707) construction
  arc A254 (-34.1909, 73.0707) -> (-37.1244, 73.1843) centre (-35.7102, 71.7701) ccw construction
  line L172 (-37.1244, 73.1843) -> (-42.4264, 67.8823) construction
  line L173 (-42.4264, 67.8823) -> (-29.746, 55.2019) construction
  line L174 (-63.6396, 46.669) -> (-44.1942, 27.2236) construction
  arc A255 (-44.1942, 27.2236) -> (-41.3657, 27.2236) centre (-42.78, 28.6378) ccw construction
  line L175 (-41.3657, 27.2236) -> (-27.2236, 41.3657) construction
  arc A256 (-27.2236, 41.3657) -> (-27.2236, 44.1942) centre (-28.6378, 42.78) ccw construction
  line L176 (-27.2236, 44.1942) -> (-46.669, 63.6396) construction
  line L177 (-46.669, 63.6396) -> (-63.6396, 46.669) construction
  line L178 (-46.669, -63.6396) -> (-27.2236, -44.1942) construction
  arc A257 (-27.2236, -44.1942) -> (-27.2236, -41.3657) centre (-28.6378, -42.78) ccw construction
  line L179 (-27.2236, -41.3657) -> (-41.3657, -27.2236) construction
  arc A258 (-41.3657, -27.2236) -> (-44.1942, -27.2236) centre (-42.78, -28.6378) ccw construction
  line L180 (-44.1942, -27.2236) -> (-63.6396, -46.669) construction
  line L181 (-63.6396, -46.669) -> (-46.669, -63.6396) construction
  arc A259 (97.9653, 2.6059) -> (90.4395, 37.7453) centre (0, 0) ccw construction
  arc A260 (90.4395, 37.7453) -> (87.1795, 38.3892) centre (88.5938, 36.975) ccw construction
  line L182 (87.1795, 38.3892) -> (83.085, 34.2947) construction
  arc A261 (76.014, 34.2947) -> (83.085, 34.2947) centre (79.5495, 37.8302) ccw construction
  line L183 (76.014, 34.2947) -> (67.8823, 42.4264) construction
  line L184 (67.8823, 42.4264) -> (47.1257, 21.6698) construction
  arc A262 (43.384, 17.9282) -> (47.1257, 21.6698) centre (43.1335, 21.9203) ccw construction
  line L185 (43.384, 17.9282) -> (26.8701, 1.4142) construction
  arc A263 (26.8701, 1.4142) -> (26.8701, -1.4142) centre (28.2843, 0) ccw construction
  line L186 (26.8701, -1.4142) -> (43.384, -17.9282) construction
  arc A264 (47.1257, -21.6698) -> (43.384, -17.9282) centre (43.1335, -21.9203) ccw construction
  line L187 (47.1257, -21.6698) -> (67.8823, -42.4264) construction
  line L188 (67.8823, -42.4264) -> (76.014, -34.2947) construction
  arc A265 (83.085, -34.2947) -> (76.014, -34.2947) centre (79.5495, -37.8302) ccw construction
  line L189 (83.085, -34.2947) -> (87.1795, -38.3892) construction
  arc A266 (87.1795, -38.3892) -> (90.4395, -37.7453) centre (88.5938, -36.975) ccw construction
  arc A267 (90.4395, -37.7453) -> (97.9653, -2.6059) centre (0, 0) ccw construction
  arc A268 (97.9653, 2.6059) -> (97.9653, -2.6059) centre (101, 0) ccw construction
  circle A269 centre (-101, 0) radius 1.6 construction
  circle A270 centre (101, 0) radius 1.6 construction
  circle A271 centre (90.3659, -45.1111) radius 1.6 construction
  circle A272 centre (-90.3659, 45.1111) radius 1.6 construction
  circle A273 centre (45.1111, -90.3659) radius 1.6 construction
  circle A274 centre (-45.1111, 90.3659) radius 1.6 construction
  circle A275 centre (90.3659, 45.1111) radius 1.6 construction
  circle A276 centre (-90.3659, -45.1111) radius 1.6 construction
  circle A277 centre (-45.1111, -90.3659) radius 1.6 construction
  circle A278 centre (45.1111, 90.3659) radius 1.6 construction
  circle A279 centre (101, 0) radius 1.6 construction
  circle A280 centre (-101, 0) radius 1.6 construction
  line L190 (101, 0) -> (-101, 0) construction
  dimension "d126" = 200.6664
  constraints: 6 end point, 4 tangent, 1 horizontal
  measures "d126" distance between parallel lines of L94 L95